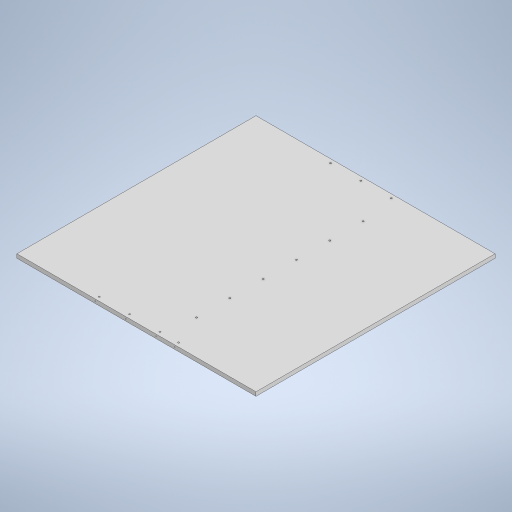
# Autodesk Inventor part: BASE
Saved by Autodesk Inventor 2023 (Build 270158000, 158)
## iProperties
Created: 2022-06-04
Part Number: BASE
Material: Generic
Document SubType Name: Modeling
Designer: prana_p9lsmih
Density: 1 g/cm^3
Appearance: Default
Author: prana_p9lsmih
Autodesk Inventor part; units mm, degrees
ref_plane "YZ Plane" through (0, 0, 0) normal (1, 0, 0) x (0, 1, 0)
ref_plane "XZ Plane" through (0, 0, 0) normal (0, 1, 0) x (-1, 0, 0)
ref_plane "XY Plane" through (0, 0, 0) normal (0, 0, 1) x (1, 0, 0)
sketch "Sketch1" plane through (0, 0, 0) normal (0, 1, 0) x (-1, 0, 0)
  line L0 (0, 0) -> (610, 0)
  line L1 (610, 0) -> (610, -610)
  line L2 (610, -610) -> (0, -610)
  line L3 (0, -610) -> (0, 0)
  dimension "d0" = 610
  dimension "d1" = 610
  constraints: 8 end point, 2 parallel, 1 horizontal, 1 perpendicular
  measures "d0" distance of L1.end L2.end
  measures "d1" distance of L0.end L1.end
extrude "Extrusion1" add sketch "Sketch1" along normal blind 10
sketch "Sketch2" plane through (-610, 0, 0) normal (0, 0, 1) x (1, 0, 0)
  line L0 (0, 0) -> (610, 0) projected
  line L1 (0, 0) -> (0, 10) projected
  point P0 (200, 5)
  dimension "d4" = 5
  dimension "d5" = 200
  measures "d4" distance from line of L0 point (200, 5)
  measures "d5" distance from line of L1 point (200, 5)
hole "Hole1" at (-410, 5, 0) direction (0, 0, -1) diameter 2 end through all
pattern_linear "Rectangular Pattern2" count 2 spacing 155 along (1, 0, 0) of "Hole1"
sketch "Sketch4" plane through (-610, 0, 0) normal (0, 0, 1) x (1, 0, 0)
  line L0 (0, 0) -> (610, 0) projected
  line L1 (610, 0) -> (610, 10) projected
  point P0 (402.5, 5)
  dimension "d28" = 5
  dimension "d29" = 207.5
  measures "d28" distance from line of L0 point (402.5, 5)
  measures "d29" distance from line of L1 point (402.5, 5)
hole "Hole3" at (-207.5, 5, 0) direction (0, 0, -1) diameter 2 depth 10 tip angle 118
pattern_linear "Rectangular Pattern3" count 2 spacing 77.5 along (1, 0, 0) of "Hole1"
sketch "Sketch5" plane through (0, 10, 0) normal (0, 1, 0) x (1, 0, 0)
  line L0 (-610, 0) -> (0, 0) projected
  line L1 (-610, 610) -> (-610, 0) projected
  point P0 (-410, 10)
  dimension "d40" = 10
  dimension "d41" = 200
  measures "d40" distance from line of L0 point (-410, 10)
  measures "d41" distance from line of L1 point (-410, 10)
hole "Hole4" at (-410, 10, -10) direction (0, -1, 0) diameter 4 end through all
pattern_linear "Rectangular Pattern4" count 3 spacing 77.5 along (1, 0, 0) of "Hole4"
sketch "Sketch6" plane through (0, 10, 0) normal (0, 1, 0) x (1, 0, 0)
  line L0 (-610, 0) -> (0, 0) projected
  line L1 (-610, 610) -> (-610, 0) projected
  point P0 (-207.5, 10)
  dimension "d52" = 10
  dimension "d53" = 402.5
  measures "d52" distance from line of L0 point (-207.5, 10)
  measures "d53" distance from line of L1 point (-207.5, 10)
hole "Hole5" at (-207.5, 10, -10) direction (0, -1, 0) diameter 4 end through all
sketch "Sketch7" plane through (0, 10, 0) normal (0, 1, 0) x (1, 0, 0)
  line L0 (0, 610) -> (-610, 610) projected
  line L1 (-610, 610) -> (-610, 0) projected
  point P0 (0, 0)
  point P1 (-410, 600)
  dimension "d61" = 10
  dimension "d62" = 200
  measures "d61" distance from line of L0 point (-410, 600)
  measures "d62" distance from line of L1 point (-410, 600)
hole "Hole6" at (-410, 10, -600) direction (0, -1, 0) diameter 4 end through all
pattern_linear "Rectangular Pattern5" count 3 spacing 77.5 along (1, 0, 0) of "Hole6"
sketch "Sketch8" plane through (0, 10, 0) normal (0, 1, 0) x (1, 0, 0)
  line L0 (0, 0) -> (0, 610) projected
  line L1 (-610, 0) -> (0, 0) projected
  point P0 (-240, 88.3)
  dimension "d73" = 240
  dimension "d74" = 88.3
  measures "d73" distance from line of L0 point (-240, 88.3)
  measures "d74" distance from line of L1 point (-240, 88.3)
hole "Hole7" at (-240, 10, -88.3) direction (0, -1, 0) diameter 4 end through all
pattern_linear "Rectangular Pattern6" count 6 spacing 85 along (0, 0, -1) of "Hole7"
body "Solid1"
